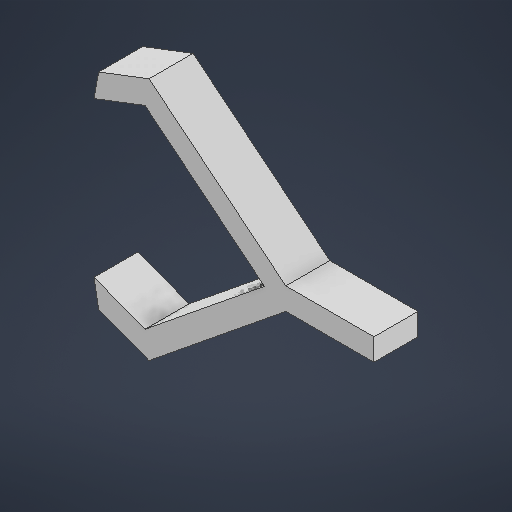
# Autodesk Inventor part: pinca
Saved by Autodesk Inventor 2026 (Build 300175050, 175E)
## iProperties
Created: 2026-04-23
Part Number: pinca
Material: Genérico
Document SubType Name: Modeling
Designer: EspacoMaker
Density: 1 g/cm^3
Appearance: Padrão
Author: EspacoMaker
Autodesk Inventor part; units mm, degrees
ref_plane "YZ Plane" through (0, 0, 0) normal (1, 0, 0) x (0, 1, 0)
ref_plane "XZ Plane" through (0, 0, 0) normal (0, 1, 0) x (-1, 0, 0)
ref_plane "XY Plane" through (0, 0, 0) normal (0, 0, 1) x (1, 0, 0)
sketch "Esboço1" plane through (0, 0, 0) normal (0, 0, 1) x (1, 0, 0)
  line L0 (-33.417, 5) -> (-95.5408, 55.4046)
  line L1 (-95.5408, 55.4046) -> (-118.417, 46.6482)
  line L2 (-118.417, 46.6482) -> (-120.5199, 35.1357)
  line L3 (-120.5199, 35.1357) -> (-97.358, 44.0015)
  line L4 (-97.358, 44.0015) -> (-22.0526, -17.098)
  line L5 (0, 0) -> (-33.417, 0)
  line L6 (-33.417, 5) -> (6.583, 5)
  line L7 (6.583, 5) -> (6.583, 0)
  line L8 (6.583, 0) -> (-33.417, 0)
  line L9 (-33.417, 0) -> (-33.417, 5)
  line L10 (-33.417, -5) -> (-95.5408, -55.4046)
  line L11 (-95.5408, -55.4046) -> (-118.417, -46.6482)
  line L12 (-118.417, -46.6482) -> (-120.5199, -35.1357)
  line L13 (-120.5199, -35.1357) -> (-97.358, -44.0015)
  line L14 (-97.358, -44.0015) -> (-22.0526, 17.098)
  line L15 (-33.417, -5) -> (6.583, -5)
  line L16 (6.583, -5) -> (6.583, 0)
  line L17 (-33.417, 0) -> (-33.417, -5)
  point P0 (-43.126, 0)
  dimension "d2" = 10
  dimension "d4" = 120
  dimension "d7" = 10
  dimension "d8" = 80
  dimension "d10" = 40
  dimension "d11" = 5
  dimension "d12" = 125
  dimension "d13" = 35.1357
  constraints: 36 end point, 7 symmetric about line, 4 parallel, 2 horizontal, 1 collinear, 1 perpendicular
  measures "d2" distance between parallel lines of L3 L1
  measures "d4" angle of L4 L3
  measures "d7" distance between parallel lines of L0 L4
  measures "d8" distance of L0.start L0.end
  measures "d10" distance of L7.end L8.end
  measures "d11" distance of L6.end L7.end
  measures "d12" horizontal distance of L6.end L1.end
  measures "d13" distance from line of L5 L2.end
extrude "Extrusão1" add sketch "Esboço1" along normal blind 20
